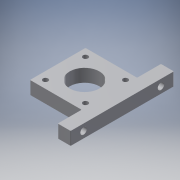
# Autodesk Inventor part: Stepper Holder X&Y_3
Saved by Autodesk Inventor 2016 (Build 200138000, 138)
## iProperties
Created: 2015-06-04
Part Number: Stepper Holder X&Y_3
Material: Aluminum 6061
Document SubType Name: Modeling
Designer: Mathias L. Kjeldgaard
Density: 2.71 g/cm^3
Appearance: Aluminum - Flat
Mass: 109.243 g
Surface Area: 120.101 cm^2
Volume: 40.3112 cm^3
Author: Mathias L. Kjeldgaard
## iProperties of the stored document Stepper Holder X&Y_3_3DPrint.ipt
Created: 2016-05-03
Part Number: Stepper Holder X&Y_3_3DPrint
Material: Generic
Document SubType Name: Modeling
Designer: Mathias L. Kjeldgaard
Appearance: Generic
Author: Mathias L. Kjeldgaard
Autodesk Inventor part; units mm, degrees
ref_plane "YZ Plane" through (0, 0, 0) normal (1, 0, 0) x (0, 1, 0)
ref_plane "XZ Plane" through (0, 0, 0) normal (0, 1, 0) x (-1, 0, 0)
ref_plane "Work Plane1" through (0, -862.1118, 0) normal (0, 0, 1) x (-1, 0, 0)
sketch "Sketch1" plane through (0, -862.1118, 0) normal (0, 0, 1) x (-1, 0, 0)
  circle A0 centre (-188, -18) radius 4 construction
  line L0 (-220, -478) -> (-220, 22) construction
  line L1 (-220, -478) -> (-208, -478) construction
  line L2 (-208, 22) -> (-208, -478) construction
  line L3 (-220, 22) -> (-208, 22) construction
  line L4 (-208, -29.2209) -> (-198, -29.2209)
  line L5 (-198, -109.2209) -> (-208, -109.2209)
  line L6 (-208, -109.2209) -> (-208, -29.2209)
  line L7 (-158, -47.7209) -> (-198, -47.7209)
  line L8 (-198, -90.7209) -> (-158, -90.7209)
  line L9 (-158, -90.7209) -> (-158, -47.7209)
  circle A1 centre (-179.15, -68.8709) radius 11.5
  circle A2 centre (-164, -53.7209) radius 2
  circle A3 centre (-195, -53.7209) radius 2
  circle A4 centre (-195, -84.7209) radius 2
  circle A5 centre (-164, -84.7209) radius 2
  line L10 (-195, -84.7209) -> (-195, -53.7209) construction
  line L11 (-195, -84.7209) -> (-164, -84.7209) construction
  line L12 (-198, -29.2209) -> (-198, -47.7209)
  line L13 (-198, -90.7209) -> (-198, -109.2209)
  point P0 (0, -862.1118)
  dimension "d0" = 10
  dimension "d1" = 80
  dimension "d3" = 43
  dimension "d4" = 18.5
  dimension "d5" = 18.5
  dimension "d6" = 23
  dimension "d7" = 4
  dimension "d8" = 4
  dimension "d9" = 4
  dimension "d10" = 4
  dimension "d11" = 31
  dimension "d12" = 31
  dimension "d13" = 31
  dimension "d14" = 31
  dimension "d15" = 6
  dimension "d18" = 6
  dimension "d19" = 6
  dimension "d20" = 6
  dimension "d21" = 90
  dimension "d25" = 21.15
  dimension "d26" = 21.15
  dimension "d27" = 90
  dimension "d28" = 90
  dimension "d29" = 18.5
  dimension "d41" = 40
  dimension "d42" = 40
  constraints: 20 end point, 5 centre point, 4 parallel, 3 perpendicular, 2 horizontal, 1 point on line
  measures "d0" distance of L5.start L5.end
  measures "d1" distance of L4.end L5.start
  measures "d3" distance between parallel lines of L8 L7
  measures "d4" distance between parallel lines of L4 L7
  measures "d5" distance between parallel lines of L5 L8
  measures "d6" diameter of A1
  measures "d7" diameter of A2
  measures "d8" diameter of A3
  measures "d9" diameter of A4
  measures "d10" diameter of A5
  measures "d11" distance of L10.end A2.centre
  measures "d12" distance of L10.start L10.end
  measures "d13" distance of L11.end L10.start
  measures "d14" distance of A2.centre L11.end
  measures "d15" distance from line of L9 A2.centre
  measures "d18" distance from line of L8 L11.end
  measures "d19" distance from line of L8 L10.start
  measures "d20" distance from line of L7 L10.end
  measures "d21" angle of L11 L10
  measures "d25" distance from line of L7 A1.centre
  measures "d26" distance from line of L9 A1.centre
  measures "d27" angle of L13 L8
  measures "d28" angle of L12 L7
  measures "d29" distance of L4.end L7.end
  measures "d41" distance of L8.start L8.end
  measures "d42" distance of L7.start L7.end
extrude "Tykkelse" add sketch "Sketch1" along normal blind 10
sketch "Sketch2" plane through (198, -832.8909, 0) normal (-1, 0, 0) x (0, 0, 1)
  line L0 (0, 0) -> (10, 0) projected
  line L1 (10, 18.5) -> (10, 0) projected
  line L2 (0, 80) -> (0, 61.5) projected
  line L3 (0, 61.5) -> (10, 61.5) projected
  line L4 (10, 80) -> (10, 61.5) projected
  line L5 (0, 80) -> (10, 80) projected
  circle A0 centre (5, 70) radius 2.5
  circle A1 centre (5, 10) radius 2.5
  point P0 (0, 832.8909)
  dimension "d32" = 5
  dimension "d33" = 5
  dimension "d34" = 10
  dimension "d35" = 5
  dimension "d36" = 5
  dimension "d37" = 10
  constraints: 2 centre point
  measures "d32" diameter of A1
  measures "d33" diameter of A0
  measures "d34" distance from line of L5 A0.centre
  measures "d35" distance from line of L4 A0.centre
  measures "d36" distance from line of L1 A1.centre
  measures "d37" distance from line of L0 A1.centre
extrude "Befæstelseshuller" cut sketch "Sketch2" against normal up to surface (10 mm away) contours A0 | A1
fillet "Fillet1" radius 0.5 8 edges at (198, -814.3909, 5) (198, -771.3909, 5) (158, -771.3909, 5) (158, -814.3909, 5) (198, -832.8909, 5) (208, -832.8909, 5) (198, -752.8909, 5) (208, -752.8909, 5)
equation "\"d4\" = d5"
equation "\"d8\" = d7"
equation "\"d9\" = d7"
equation "\"d10\" = d7"
equation "\"d13\" = d11"
equation "\"d14\" = d12"
equation "\"d15\" = d20"
equation "\"d18\" = d15"
equation "\"d19\" = d18"
equation "\"d42\" = d41"
equation "\"d32\" = d33"
equation "\"d36\" = d35"
equation "\"d37\" = d34"
body "Solid1"
